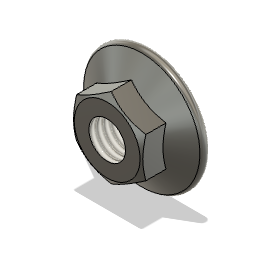
Motor_Mount v5 (Autodesk Fusion 360 archive; units mm, degrees)
design "Hex Flange Nut ANSI B18.2.4.4M - M5 x 0.8 Steel Grade 8 Plain"
description: Hex Flange Nut ANSI B18.2.4.4M - M5 x 0.8
Autodesk Fusion 360 part; units mm, degrees
sketch "Sketch1" plane through (0, 0, 0) normal (0, 1, 0) x (1, 0, 0)
  line L0 (0, 0) -> (0, -5)
  line L1 (-2.5, 0) -> (-4.62, 0)
  line L2 (-4.62, 0) -> (-4.62, -4.5266)
  line L3 (-3.8, -5) -> (-2.5, -5)
  line L4 (-4.62, -4.5266) -> (-3.8, -5)
  line L5 (-2.5, -5) -> (-2.5, 0)
  dimension "d81" = 9.24
  dimension "d149" = 5
  dimension "d150" = 30
  dimension "d151" = 7.6
  dimension "d152" = 5
  constraint coincident L0.start L1
  constraint vertical L0
  constraint parallel L0 L2
  constraint coincident L0 L0.end
  constraint perpendicular L0 L3
  constraint perpendicular L0 L1
  constraint coincident origin L0
  constraint coincident L0.start origin
  constraint perpendicular L1 L5
  constraint coincident L0.end L3
  measures "d149" distance of L1 L3
  measures "d150" angle of L3 L4
revolve "Revolve1" add sketch "Sketch1" angle 360 about axis through (0, 0, 0) along (0, 0, 1)
sketch "Sketch8" plane through (0, 0, 5) normal (0, 0, 1) x (1, 0, 0)
  line L0 (0, 0) -> (-8, 0) construction
  line L1 (-4, -2.3118) -> (-4, 2.3118)
  circle A0 centre (0, 0) radius 3.8
  circle A1 centre (0, 0) radius 4.62
  circle A2 centre (0, 0) radius 2.5
  dimension "d121" = 4
  constraint horizontal L0
  constraint perpendicular L0 L1
  constraint midpoint L0 L1
  constraint coincident L1.end A1
  constraint coincident L1.start A1
  constraint coincident L0.start A0.centre
  measures "d121" distance of L0.start L1
extrude "Extrude5" cut sketch "Sketch8" against normal blind 5 contours L1 A1 picked at (-4.1, -0.5631)
pattern_circular "C-Pattern2" count 6 over 360 about axis through (0, 0, 1.75) along (0, 0, 1) of "Extrude5"
thread "Thread4" "ANSI Metric M Profile 5.0 M5x0.8 6H" major diameter 5.12 minor diameter 4.234 pitch 0.8 angle 60 resizes the face on face at (-2.4876, 0.2489, 3.3333)
sketch "Sketch12" plane through (0, 0, 0) normal (1, 0, 0) x (0, 0, -1)
  line L0 (-1, 6.7038) -> (-3.4271, 2.5)
  line L1 (-3.4271, 2.5) -> (0, 2.5)
  arc A0 (0, 6.4359) -> (-1, 6.7038) centre (-0.5359, 6.4359) ccw
  line L2 (-0.5359, 6.4359) -> (-0.5359, 5.9) construction
  line L3 (0, 0) -> (-5, 0)
  line L4 (0, 6.4359) -> (0, 0)
  dimension "d145" = 5
  dimension "d146" = 11.8
  dimension "d147" = 1
  dimension "d148" = 30
  constraint tangent L0 A0
  constraint coincident A0.centre L2.start
  constraint coincident A0 L2.end
  constraint coincident L3.start L4.end
  constraint tangent A0 L4
  constraint coincident L1.end L4
  constraint vertical L2
  constraint perpendicular L1 L4
  constraint perpendicular L3 L4
  measures "d145" distance of L1.end L3
  measures "d147" horizontal distance of A0.start L0.start
  measures "d148" angle of L0 L4
revolve "Revolve3" add sketch "Sketch12" angle 360 about axis through (0, 0, 1.75) along (0, 0, 1)
equation "adsk_nheig = 5.00 mm"
equation "adsk_wacor = 9.24 mm"
equation "adsk_nomdia = 5.00 mm"
equation "d81 = adsk_wacor"
equation "d89 = -adsk_nheig"
equation "adsk_waflat = 8.00 mm"
equation "adsk_maxdia = 11.80 mm"
equation "adsk_flngheig = 1.00 mm"
equation "d121 = adsk_waflat / 2"
equation "adsk_chamang2 = 30.00 deg"
equation "adsk_flngang = 30.00 deg"
equation "d143 = adsk_nheig"
equation "d145 = adsk_nomdia"
equation "d146 = adsk_maxdia"
equation "d147 = adsk_flngheig"
equation "d148 = adsk_flngang"
equation "d149 = adsk_nheig"
equation "d150 = adsk_chamang2"
equation "d151 = adsk_waflat * 0.95"
equation "d152 = adsk_nomdia"

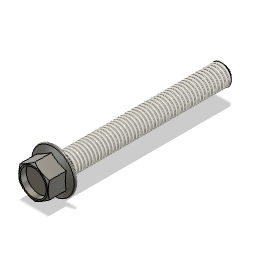
design "Indented Hex Flange Head Machine Screw ANSI B18.6.7M - M5x0.8 x 40 Steel Grade 8 Plain"
description: Indented Hex Flange Head Machine Screw ANSI B18.6.7M - M5x0.8 x 40
Autodesk Fusion 360 part; units mm, degrees
sketch "Sketch1" plane through (0, 0, 0) normal (0, 1, 0) x (1, 0, 0)
  line L0 (-2.5, 0) -> (-2.5, 40)
  line L1 (-2.5, 40) -> (0, 40)
  line L2 (0, 40) -> (0, -4)
  line L3 (-2.5, 0) -> (-4.0425, 0)
  line L4 (-4.0425, 0) -> (-4.0425, -5.0464)
  line L5 (-3.43, -5.4) -> (-3.1, -5.4)
  line L6 (-3.43, -5.4) -> (-4.0425, -5.0464)
  line L7 (-3.1, -5.4) -> (-3.1, -4)
  line L8 (-3.1, -4) -> (0, -4)
  dimension "d9" = 5
  dimension "d68" = 40
  dimension "d111" = 5.4
  dimension "d113" = 30
  dimension "d114" = 8.085
  dimension "d115" = 6.86
  dimension "d158" = 6.2
  dimension "d159" = 1.4
  constraint perpendicular L0 L1
  constraint perpendicular L0 L3
  constraint coincident origin L3
  constraint vertical L0
  constraint vertical L2
  constraint parallel L2 L4
  constraint coincident L2 L8.end
  constraint perpendicular L2 L5
  constraint coincident L3.end L4.start
  constraint perpendicular L5 L7
  constraint perpendicular L2 L8
  constraint coincident L2.end L8.end
  constraint coincident origin L2
  measures "d68" distance of origin L1.end
  measures "d111" distance of L3 L5
  measures "d113" angle of L5 L6
  measures "d159" distance of L5.end L7.end
revolve "Revolve1" add sketch "Sketch1" angle 360 about axis through (0, 0, -40) along (0, 0, 1)
sketch "Sketch8" plane through (0, 0, 0) normal (0, 0, 1) x (1, 0, 0)
  line L0 (0, 0) -> (-3.5, 0) construction
  line L1 (-3.5, -2.0228) -> (-3.5, 2.0228)
  circle A0 centre (0, 0) radius 4.0425
  dimension "d110" = 3.5
  constraint horizontal L0
  constraint perpendicular L0 L1
  constraint coincident L0.end L1
  constraint coincident L0.start A0.centre
  constraint coincident L1.end A0
  constraint coincident L1.start A0
  measures "d110" distance of L0.start L1
extrude "Extrude5" cut sketch "Sketch8" along normal blind 5.4 contours L1 A0 picked at (-3.5875, -0.4927)
pattern_circular "C-Pattern2" count 6 over 360 about axis through (0, 0, 1.75) along (0, 0, 1) of "Extrude5"
sketch "Sketch12" plane through (0, 0, 0) normal (0, 1, 0) x (1, 0, 0)
  line L0 (3.325, 0) -> (4.9391, 0)
  line L1 (5.0625, -0.7) -> (3.325, -1.3324)
  line L2 (3.325, -1.3324) -> (3.325, 0)
  arc A0 (5.0625, -0.7) -> (4.9391, 0) centre (4.9391, -0.3609) ccw
  line L3 (0, -1.75) -> (0, -22.5)
  line L4 (4.0425, 0) -> (4.0425, -1.0713) construction
  line L5 (0, 0) -> (3.5, 0)
  line L6 (5.3, 0) -> (5.3, -1.3324) construction
  line L7 (3.325, -1.3324) -> (5.3, -1.3324) construction
  dimension "d122" = 6.65
  dimension "d126" = 8.085
  dimension "d138" = 0.7
  dimension "d142" = 5.3
  dimension "d163" = 20
  constraint horizontal L0
  constraint perpendicular L0 L2
  constraint tangent L0 A0
  constraint tangent L1 A0
  constraint horizontal L5.start L0.start
  constraint coincident L1 L4.end
  constraint perpendicular L0 L4
  constraint coincident L0 L4.start
  constraint vertical L6
  constraint tangent A0 L6
  constraint coincident L0 L6.start
  constraint perpendicular L6 L7
  constraint coincident L6.end L7.end
  measures "d138" vertical distance of L0.end L1.start
  measures "d142" distance of L5.start L6
  measures "d163" angle of L0 L1
revolve "Revolve3" add sketch "Sketch12" angle 360 about axis through (0, 0, 1.75) along (0, 0, 1)
thread "Thread2" "ISO Metric profile 5.0 M5x0.8 6g" major diameter 4.901 minor diameter 3.9895 pitch 0.8 angle 60 resizes the face on face at (-2.4876, 0.2489, -13.3333) from (0, 0, -1.8) to (0, 0, -40)
fillet "Fillet4" radius 0.1667 1 edges at (2.2847, -0.8861, 0)
sketch "Sketch5" plane through (0, 0, 0) normal (0, 1, 0) x (1, 0, 0)
  line L0 (-2.55, 39.3) -> (-1.8, 40)
  line L1 (0, -1.75) -> (0, -22.5)
  line L2 (0, 40) -> (0, -4)
  line L3 (0, 40) -> (-2.55, 40)
  line L4 (-2.55, 40) -> (-2.55, 39.3)
  dimension "d153" = 1.8
  dimension "d156" = 2.55
  dimension "d157" = 0.7
  constraint coincident L2.start L3.start
  constraint perpendicular L2 L3
  constraint coincident L0.end L3
  constraint perpendicular L3 L4
  measures "d153" distance of L0.end L1
  measures "d156" horizontal distance of origin L3.end
  measures "d157" distance of L0.start L3.end
revolve "Revolve2" cut sketch "Sketch5" angle 360 about axis through (0, 0, -40) along (0, 0, 1)
equation "d9 = adsk_nomdia"
equation "adsk_nomlen = 40.00 mm"
equation "adsk_headh = 5.40 mm"
equation "adsk_nomdia = 5.00 mm"
equation "d68 = adsk_nomlen"
equation "d89 = adsk_headh"
equation "adsk_waflat = 7.00 mm"
equation "d110 = adsk_waflat / 2"
equation "d111 = adsk_headh"
equation "d113 = adsk_chamang2"
equation "d114 = adsk_wacor"
equation "d115 = adsk_topdia"
equation "d122 = adsk_waflat * 0.95"
equation "d126 = adsk_waflat * 1.155"
equation "adsk_headdia = 10.60 mm"
equation "adsk_flngheig = 0.70 mm"
equation "adsk_thrlen = 38.20 mm"
equation "d133 = adsk_nomdia / 30"
equation "d138 = adsk_flngheig"
equation "d142 = adsk_headdia / 2"
equation "d144 = adsk_thrlen"
equation "adsk_endpointdia = 3.60 mm"
equation "d153 = adsk_endpointdia / 2"
equation "adsk_startlen = 0.70 mm"
equation "d156 = adsk_nomdia * 0.51"
equation "d157 = adsk_startlen"
equation "d158 = adsk_indentdia"
equation "d159 = adsk_indentdepth"
equation "adsk_wacor = 8.085 mm"
equation "adsk_topdia = adsk_waflat * 0.98"
equation "adsk_chamang2 = 30.00 deg"
equation "d163 = adsk_flngang"
equation "adsk_flngang = 20.00 deg"
equation "adsk_indentdia = 6.20 mm"
equation "adsk_indentdepth = 1.40 mm"
